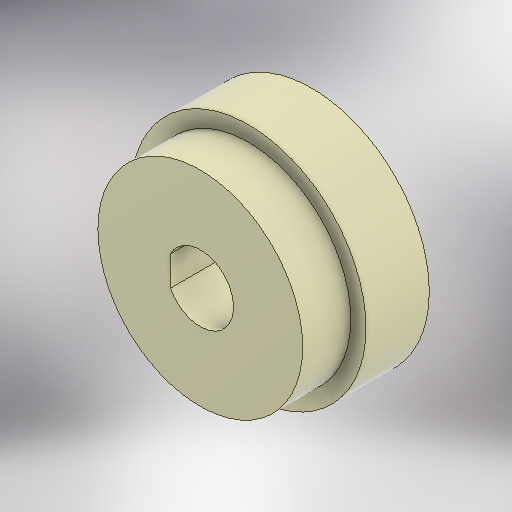
# Autodesk Inventor part: wheel_mount
Saved by Autodesk Inventor 2026 (Build 300175050, 175E)
## iProperties
Created: 2025-06-04
Part Number: wheel_mount
Material: Generic
Document SubType Name: Modeling
Designer: satom
Density: 1 g/cm^3
Appearance: Smooth - Ash
Author: satom
Autodesk Inventor part; units mm, degrees
ref_plane "YZ Plane" through (0, 0, 0) normal (1, 0, 0) x (0, 1, 0)
ref_plane "XZ Plane" through (0, 0, 0) normal (0, 1, 0) x (-1, 0, 0)
ref_plane "XY Plane" through (0, 0, 0) normal (0, 0, 1) x (1, 0, 0)
sketch "Sketch1" plane through (0, 0, 0) normal (0, 0, 1) x (1, 0, 0)
  circle A0 centre (0, 0) radius 10.85
  dimension "d0" = 21.7
  constraints: 1 centre point, 1 coincident
  measures "d0" diameter of A0
extrude "Extrusion1" add sketch "Sketch1" along normal blind 5.842
sketch "Sketch2" plane through (0, 0, 5.842) normal (0, 0, 1) x (1, 0, 0)
  circle A0 centre (0, 0) radius 9.45
  dimension "d3" = 18.9
  constraints: 1 centre point, 1 coincident
  measures "d3" diameter of A0
extrude "Extrusion2" add sketch "Sketch2" along normal blind 4.445
sketch "Sketch3" plane through (0, 0, 10.287) normal (0, 0, 1) x (1, 0, 0)
  circle A0 centre (0, 0) radius 3.075
  circle A1 centre (0, 0) radius 10.85 construction
  line L0 (-10.85, 0) -> (10.85, 0) construction
  circle A2 centre (0, 0) radius 9.45 construction
  line L1 (0, 9.45) -> (0, -9.45) construction
  line L2 (-2.75, 1.3759) -> (-2.75, -1.3759)
  dimension "d13" = 6.15
  dimension "d16" = 2.75
  constraints: 6 end point, 6 point on circle, 2 horizontal, 2 midpoint, 1 centre point, 1 coincident, 1 perpendicular, 1 vertical, 1 other
  measures "d13" diameter of A0
  measures "d16" distance from line of A0.centre L2
extrude "Extrusion3" cut sketch "Sketch3" against normal through all contours A0 L2 picked at (-0.8083, 0)
body "Solid1"
